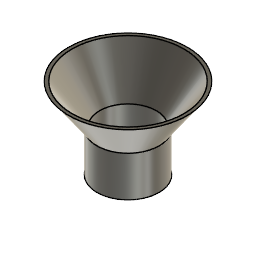
Trichter (Autodesk Fusion 360 design; units mm, degrees)
Autodesk Fusion 360 part; units mm, degrees
cylinder "Grundkörper Zylinder1" add diameter 23 height 15 placed x (1, 0, 0) y (0, 1, 0) z (0, 0, 1) at (0, 0, 0) makes body 1
cylinder "Grundkörper Zylinder2" add diameter 23 height 15 placed x (1, 0, 0) y (0, 1, 0) z (0, 0, 1) at (0, 0, 15) separate body makes body 2
draft "Verjüngung1" angle 35 neutral plane through (0, 0, 15) pull (0, 0, -1) 1 faces at (11.4429, -1.145, 20) on bodies 2
combine "Kombinieren1" operation add target body 1 tool bodies 2
shell "Schale1" thickness 1 removed faces 2 at (3.663, 4.0848, 0) at (-0.4395, 6.8382, 30) on bodies 1
